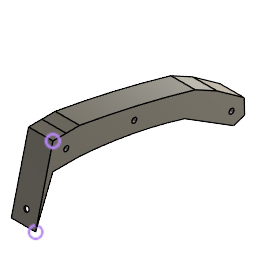
Arm v2 (Autodesk Fusion 360 design; units mm, degrees)
Autodesk Fusion 360 part; units mm, degrees
sketch "Sketch1" plane through (0, 0, 0) normal (1, 0, 0) x (0, 1, 0)
  circle A0 centre (0, 0) radius 2.6
  circle A1 centre (175.9096, -53.4375) radius 2.6
  line L0 (137.2781, -14.356) -> (160.424, -26.9456)
  line L1 (160.424, -26.9456) -> (189.4776, -47.6848)
  line L2 (189.4776, -47.6848) -> (189.9997, -63.9991)
  line L3 (189.9997, -63.9991) -> (178.1831, -67.9555)
  line L4 (178.1831, -67.9555) -> (125.9198, -35.3622)
  circle A2 centre (72.465, -10.0775) radius 2.6
  line L5 (-14.2, 14.2002) -> (-32.5668, -60.5772)
  line L6 (0, 14.2002) -> (14.2, 14.3859)
  line L7 (0, 14.2002) -> (-14.2, 14.2002)
  line L8 (0, -14.2002) -> (14.2, -14.2002)
  line L9 (0, -14.2002) -> (-14.2, -14.2002)
  line L10 (-14.2, -14.2002) -> (-32.5668, -60.5772)
  arc A3 (137.2781, -14.356) -> (14.2, 14.3859) centre (-186.9778, -1124.9865) ccw
  arc A4 (125.9198, -35.3622) -> (14.2, -14.2002) centre (-22.4488, -513.1589) ccw
  dimension "d1" = 5.2
  dimension "d7" = 5.2
  dimension "d37" = 5.2
  dimension "d40" = 77
  constraint coincident A0.centre origin
  measures "d1" diameter of A0
  measures "d7" diameter of A1
  measures "d37" diameter of A2
  measures "d40" distance of L5.end L5.start
extrude "Extrude1" add sketch "Sketch1" along normal mid plane 52
sketch "Sketch2" plane through (0, -16.6815, 4.0973) normal (0, -0.971135, 0.23853) x (1, 0, 0)
  line L0 (26, -66.5968) -> (26, 10.4032)
extrude "Extrude2" cut 1 faces at (-26, 27.9887, 2.1627) along direction (1, 0, 0) blind 26
sketch "Sketch3" plane through (0, -16.6815, 4.0973) normal (0, -0.971135, 0.23853) x (1, 0, 0)
  line L0 (0, 10.4032) -> (0, -66.5968)
  line L1 (0, -66.5968) -> (26, -66.5968)
  line L2 (26, -66.5968) -> (26, 10.4032)
  line L3 (26, 10.4032) -> (0, 10.4032)
  circle A0 centre (13, -53.0968) radius 2.6
  dimension "d53" = 5.2
  measures "d53" diameter of A0
extrude "Extrude3" cut sketch "Sketch3" against normal blind 5 contours A0
